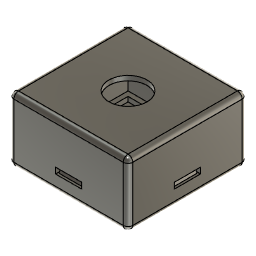
Button_case (Autodesk Fusion 360 design; units mm, degrees)
Autodesk Fusion 360 part; units mm, degrees
note: some values were not read from the file. Set by a fixed rule: which sketch regions a step uses.
sketch "Sketch1" plane through (0, 0, 0) normal (0, 0, 1) x (1, 0, 0)
  line L0 (0, 0) -> (50, 0)
  line L1 (50, 0) -> (50, 50)
  line L2 (50, 50) -> (0, 50)
  line L3 (0, 50) -> (0, 0)
  circle A0 centre (25, 25) radius 8
  line L4 (2, 48) -> (48, 48)
  line L5 (48, 48) -> (48, 2)
  line L6 (48, 2) -> (2, 2)
  line L7 (2, 2) -> (2, 48)
  constraint horizontal L0
  constraint vertical L1
  constraint horizontal L2
  constraint vertical L3
  constraint coincident L0.start L3.end
  constraint horizontal L4
  constraint vertical L5
  constraint horizontal L6
  constraint vertical L7
extrude "Extrude1" add sketch "Sketch1" along normal blind 2 contours L0 L1 L2 L3 | L4 L5 L6 L7 makes body 1
extrude "Extrude2" add sketch "Sketch1" against normal blind 23 contours L0 L1 L2 L3 bodies 1
fillet "Fillet1" radius 2 8 edges at (0, 25, 2) (25, 0, 2) (25, 50, 2) (50, 25, 2) (0, 0, -10.5) (50, 0, -10.5) (50, 50, -10.5) (0, 50, -10.5) on bodies 1
sketch "Sketch2" plane through (0, 0, -23) normal (0, 0, -1) x (1, 0, 0)
  arc A0 (50, -2) -> (48, 0) centre (48, -2) ccw
  line L0 (48, 0) -> (2, 0)
  arc A1 (2, 0) -> (0, -2) centre (2, -2) ccw
  line L1 (0, -2) -> (0, -48)
  arc A2 (0, -48) -> (2, -50) centre (2, -48) ccw
  line L2 (2, -50) -> (48, -50)
  arc A3 (48, -50) -> (50, -48) centre (48, -48) ccw
  line L3 (50, -48) -> (50, -2)
  line L4 (2, -2) -> (48, -2)
  line L5 (48, -2) -> (48, -48)
  line L6 (48, -48) -> (2, -48)
  line L7 (2, -48) -> (2, -2)
  line L8 (0, 0) -> (50, 0)
  line L9 (50, 0) -> (50, -50)
  line L10 (50, -50) -> (0, -50)
  line L11 (0, -50) -> (0, 0)
  line L12 (2, -2) -> (48, -2)
  line L13 (48, -2) -> (48, -48)
  line L14 (48, -48) -> (2, -48)
  line L15 (2, -48) -> (2, -2)
  line L16 (4, -46) -> (46, -46)
  line L17 (46, -46) -> (46, -4)
  line L18 (46, -4) -> (4, -4)
  line L19 (4, -4) -> (4, -46)
  constraint horizontal L8
  constraint vertical L9
  constraint horizontal L10
  constraint vertical L11
  constraint coincident L8.start L11.end
  constraint horizontal L12
  constraint vertical L13
  constraint horizontal L14
  constraint vertical L15
  constraint coincident A3.centre L5.end
  constraint coincident A1.centre L4.start
  constraint horizontal L16
  constraint vertical L17
  constraint horizontal L18
  constraint vertical L19
extrude "Extrude3" add sketch "Sketch2" along normal blind 2 separate body contours A0 L0 A1 L1 A2 L2 A3 L3 L8 L9 L10 L11 | L4 L5 L6 L7 L12 L13 L14 L15 | L16 L17 L18 L19 makes body 2
fillet "Fillet2" radius 2 8 edges at (50, 25, -25) (49.4142, 0.5858, -25) (25, 0, -25) (0.5858, 0.5858, -25) (0, 25, -25) (0.5858, 49.4142, -25) (25, 50, -25) (49.4142, 49.4142, -25) on bodies 2
extrude "Extrude4" add sketch "Sketch2" against normal blind 2 contours L4 L5 L6 L7 L12 L13 L14 L15 bodies 2
sketch "Sketch3" plane through (0, 0, -21) normal (0, 0, 1) x (-1, 0, 0)
  line L0 (-4, -4) -> (-4, -46)
  line L1 (-4, -46) -> (-46, -46)
  line L2 (-46, -46) -> (-46, -4)
  line L3 (-46, -4) -> (-4, -4)
  line L4 (-48, -48) -> (-2, -48)
  line L5 (-2, -48) -> (-2, -2)
  line L6 (-2, -2) -> (-48, -2)
  line L7 (-48, -2) -> (-48, -48)
  line L8 (-4, -30) -> (-2, -30)
  line L9 (-2, -30) -> (-2, -19.9838)
  line L10 (-2, -19.9838) -> (-4, -19.9838)
  line L11 (-4, -19.9838) -> (-4, -30)
  line L12 (-20, -46) -> (-30.0621, -46)
  line L13 (-30.0621, -46) -> (-30.0621, -48)
  line L14 (-30.0621, -48) -> (-20, -48)
  line L15 (-20, -48) -> (-20, -46)
  line L16 (-46, -30) -> (-48, -30)
  line L17 (-48, -30) -> (-48, -19.979)
  line L18 (-48, -19.979) -> (-46, -19.979)
  line L19 (-46, -19.979) -> (-46, -30)
  line L20 (-20, -4) -> (-30.0621, -4)
  line L21 (-30.0621, -4) -> (-30.0621, -2)
  line L22 (-30.0621, -2) -> (-20, -2)
  line L23 (-20, -2) -> (-20, -4)
  constraint horizontal L8
  constraint vertical L9
  constraint horizontal L10
  constraint vertical L11
  constraint coincident L5 L9.end
  constraint coincident L0 L8.start
  constraint horizontal L12
  constraint vertical L13
  constraint horizontal L14
  constraint vertical L15
  constraint coincident L4 L13.end
  constraint coincident L1 L12.start
  constraint horizontal L16
  constraint vertical L17
  constraint horizontal L18
  constraint vertical L19
  constraint coincident L7 L17.end
  constraint coincident L2 L16.start
  constraint horizontal L20
  constraint vertical L21
  constraint horizontal L22
  constraint vertical L23
  constraint coincident L6 L21.end
  constraint coincident L3 L20.start
extrude "Extrude5" add sketch "Sketch3" along normal blind 5 contours L0 L5 L8 L9 L10 L11 bodies 2
sketch "Sketch4" plane through (2, 0, 0) normal (-1, 0, 0) x (0, -1, 0)
  line L0 (-48, -23) -> (-2, -23)
  line L1 (-2, -23) -> (-2, -21)
  line L2 (-2, -21) -> (-19.9838, -21)
  line L3 (-19.9838, -21) -> (-19.9838, -16)
  line L4 (-19.9838, -16) -> (-30, -16)
  line L5 (-30, -16) -> (-30, -21)
  line L6 (-30, -21) -> (-48, -21)
  line L7 (-48, -21) -> (-48, -23)
  line L8 (-30, -16) -> (-19.9838, -16)
  line L9 (-19.9838, -16) -> (-19.9838, -18.5)
  line L10 (-19.9838, -18.5) -> (-30, -18.5)
  line L11 (-30, -18.5) -> (-30, -16)
  constraint horizontal L8
  constraint vertical L9
  constraint horizontal L10
  constraint vertical L11
  constraint midpoint L3 L9.end
  constraint coincident L4.end L5.start
extrude "Extrude6" add sketch "Sketch4" along normal blind 2 contours L3 L4 L5 L8 L9 L10 L11 bodies 2
sketch "Sketch5" plane through (0, 30, 0) normal (0, 1, 0) x (-1, 0, 0)
  line L0 (-4, -21) -> (-2, -21)
  line L1 (-2, -21) -> (-2, -18.5)
  line L2 (-2, -18.5) -> (0, -18.5)
  line L3 (0, -18.5) -> (0, -16)
  line L4 (0, -16) -> (-4, -16)
  line L5 (-4, -16) -> (-4, -21)
  line L6 (0, -18.5) -> (0, -17.5)
  line L7 (0, -17.5) -> (-2, -16)
  line L8 (0, -18.5) -> (-1, -18.5)
  line L9 (-1, -18.5) -> (-2, -16)
  constraint coincident L2.end L3.start
  constraint coincident L3 L6.end
  constraint perpendicular L2 L6
  constraint midpoint L4 L7.end
  constraint midpoint L2 L8.end
extrude "Extrude7" cut sketch "Sketch5" against normal blind 28 contours L3 L4 L7 bodies 2
copy_body "CopyPasteBodies1" bodies 2 makes body 3
move_body "Move1" bodies 3 to x (1, 0, 0) y (0, 1, 0) z (0, 0, 1) at (0, 0, 0)
combine "Combine1" operation cut target body 1 tool bodies 3
extrude "Extrude8" add sketch "Sketch3" along normal blind 5 contours L3 L6 L20 L21 L22 L23 | L1 L4 L12 L13 L14 L15 | L2 L7 L16 L17 L18 L19 bodies 2
sketch "Sketch6" plane through (0, 2, 0) normal (0, -1, 0) x (1, 0, 0)
  line L0 (2, -23) -> (48, -23)
  line L1 (48, -23) -> (48, -21)
  line L2 (48, -21) -> (30.0621, -21)
  line L3 (30.0621, -21) -> (30.0621, -16)
  line L4 (30.0621, -16) -> (20, -16)
  line L5 (20, -16) -> (20, -21)
  line L6 (20, -21) -> (2, -21)
  line L7 (2, -21) -> (2, -23)
  line L8 (20, -16) -> (30.0621, -16)
  line L9 (30.0621, -16) -> (30.0621, -18.5)
  line L10 (30.0621, -18.5) -> (20, -18.5)
  line L11 (20, -18.5) -> (20, -16)
  constraint horizontal L8
  constraint vertical L9
  constraint horizontal L10
  constraint vertical L11
  constraint midpoint L3 L9.end
  constraint coincident L4.end L5.start
extrude "Extrude9" add sketch "Sketch6" along normal blind 2 contours L3 L4 L5 L8 L9 L10 L11 bodies 2
sketch "Sketch7" plane through (20, 0, 0) normal (-1, 0, 0) x (0, -1, 0)
  line L0 (-4, -21) -> (-2, -21)
  line L1 (-2, -21) -> (-2, -18.5)
  line L2 (-2, -18.5) -> (0, -18.5)
  line L3 (0, -18.5) -> (0, -16)
  line L4 (0, -16) -> (-4, -16)
  line L5 (-4, -16) -> (-4, -21)
  line L6 (-2, -16) -> (0, -17.5)
  line L7 (0, -18.5) -> (-1, -18.5)
  line L8 (-2, -16) -> (-1, -18.5)
  constraint midpoint L4 L6.start
  constraint coincident L3 L6.end
  constraint coincident L2.end L3.start
  constraint midpoint L2 L7.end
extrude "Extrude10" cut sketch "Sketch7" against normal blind 42 contours L3 L4 L6 bodies 2
sketch "Sketch8" plane through (0, 48, 0) normal (0, 1, 0) x (-1, 0, 0)
  line L0 (-48, -23) -> (-2, -23)
  line L1 (-2, -23) -> (-2, -21)
  line L2 (-2, -21) -> (-20, -21)
  line L3 (-20, -21) -> (-20, -16)
  line L4 (-20, -16) -> (-30.0621, -16)
  line L5 (-30.0621, -16) -> (-30.0621, -21)
  line L6 (-30.0621, -21) -> (-48, -21)
  line L7 (-48, -21) -> (-48, -23)
  line L8 (-30.0621, -16) -> (-20, -16)
  line L9 (-20, -16) -> (-20, -18.5)
  line L10 (-20, -18.5) -> (-30.0621, -18.5)
  line L11 (-30.0621, -18.5) -> (-30.0621, -16)
  constraint horizontal L8
  constraint vertical L9
  constraint horizontal L10
  constraint vertical L11
  constraint midpoint L3 L9.end
  constraint coincident L4.end L5.start
extrude "Extrude11" add sketch "Sketch8" along normal blind 2 contours L3 L4 L5 L8 L9 L10 L11 bodies 2
sketch "Sketch9" plane through (30.0621, 0, 0) normal (1, 0, 0) x (0, 1, 0)
  line L0 (46, -21) -> (48, -21)
  line L1 (48, -21) -> (48, -18.5)
  line L2 (48, -18.5) -> (50, -18.5)
  line L3 (50, -18.5) -> (50, -16)
  line L4 (50, -16) -> (46, -16)
  line L5 (46, -16) -> (46, -21)
  line L6 (48, -16) -> (50, -17.5)
  line L7 (50, -18.5) -> (49, -18.5)
  line L8 (48, -16) -> (49, -18.5)
  constraint midpoint L4 L6.start
  constraint coincident L3 L6.end
  constraint coincident L2.end L3.start
  constraint midpoint L2 L7.end
extrude "Extrude12" cut sketch "Sketch9" against normal blind 37 contours L3 L4 L6 bodies 2
sketch "Sketch10" plane through (48, 0, 0) normal (1, 0, 0) x (0, 1, 0)
  line L0 (2, -23) -> (48, -23)
  line L1 (48, -23) -> (48, -21)
  line L2 (48, -21) -> (30, -21)
  line L3 (30, -21) -> (30, -16)
  line L4 (30, -16) -> (19.979, -16)
  line L5 (19.979, -16) -> (19.979, -21)
  line L6 (19.979, -21) -> (2, -21)
  line L7 (2, -21) -> (2, -23)
  line L8 (19.979, -16) -> (30, -16)
  line L9 (30, -16) -> (30, -18.5)
  line L10 (30, -18.5) -> (19.979, -18.5)
  line L11 (19.979, -18.5) -> (19.979, -16)
  constraint horizontal L8
  constraint vertical L9
  constraint horizontal L10
  constraint vertical L11
  constraint midpoint L3 L9.end
  constraint coincident L4.end L5.start
extrude "Extrude13" add sketch "Sketch10" along normal blind 2 contours L3 L4 L5 L8 L9 L10 L11 bodies 2
sketch "Sketch11" plane through (0, 19.979, 0) normal (0, -1, 0) x (1, 0, 0)
  line L0 (46, -21) -> (48, -21)
  line L1 (48, -21) -> (48, -18.5)
  line L2 (48, -18.5) -> (50, -18.5)
  line L3 (50, -18.5) -> (50, -16)
  line L4 (50, -16) -> (46, -16)
  line L5 (46, -16) -> (46, -21)
  line L6 (48, -16) -> (50, -17.5)
  line L7 (50, -18.5) -> (49, -18.5)
  line L8 (49, -16.75) -> (49, -18.5)
  line L9 (48, -16) -> (49, -18.5)
  constraint midpoint L4 L6.start
  constraint coincident L3 L6.end
  constraint coincident L2.end L3.start
  constraint midpoint L2 L7.end
  constraint midpoint L6 L8.start
extrude "Extrude14" cut sketch "Sketch11" against normal blind 23 contours L3 L4 L6 bodies 2
copy_body "CopyPasteBodies2" bodies 2 makes body 4
move_body "Move2" bodies 4 to x (1, 0, 0) y (0, 1, 0) z (0, 0, 1) at (0, 0, 0)
combine "Combine2" operation cut target body 1 tool bodies 4
sketch "Sketch12" plane through (0, 0, 0) normal (-1, 0, 0) x (0, -1, 0)
  line L0 (-30, -17.5) -> (-19.9838, -17.5)
  line L1 (-19.9838, -17.5) -> (-19.9838, -18.5)
  line L2 (-19.9838, -18.5) -> (-30, -18.5)
  line L3 (-30, -18.5) -> (-30, -17.5)
  line L4 (-2, -23) -> (-2, 0)
  line L5 (-2, 0) -> (-48, 0)
  line L6 (-48, 0) -> (-48, -23)
  line L7 (-48, -23) -> (-2, -23)
  line L8 (-30, -18.5) -> (-30.5, -18.5)
  line L9 (-30.5, -18.5) -> (-30.5, -19)
  line L10 (-19.9838, -18.5) -> (-19.5, -18.5)
  line L11 (-19.5, -18.5) -> (-19.5, -19)
  line L12 (-19.5, -19) -> (-30.5, -19)
  line L13 (-30.5, -19) -> (-30.5, -16)
  line L14 (-30.5, -16) -> (-19.5, -16)
  line L15 (-19.5, -16) -> (-19.5, -18.5)
  line L16 (-19.9838, -18.5) -> (-19.5, -18.5)
  line L17 (-30, -18.5) -> (-30.5, -18.5)
  constraint coincident L2.end L3.start
  constraint perpendicular L3 L8
  constraint perpendicular L8 L9
  constraint coincident L1.end L2.start
  constraint perpendicular L1 L10
  constraint perpendicular L10 L11
  constraint perpendicular L8 L13
  constraint perpendicular L13 L14
  constraint perpendicular L10 L15
extrude "Extrude15" cut sketch "Sketch12" against normal blind 84 contours L0 L1 L3 L8 L10 L13 L14 L15 L16 L17 bodies 1
sketch "Sketch13" plane through (0, 50, 0) normal (0, 1, 0) x (-1, 0, 0)
  line L0 (-30.0621, -17.5) -> (-20, -17.5)
  line L1 (-20, -17.5) -> (-20, -18.5)
  line L2 (-20, -18.5) -> (-30.0621, -18.5)
  line L3 (-30.0621, -18.5) -> (-30.0621, -17.5)
  line L4 (-48, 0) -> (-48, -23)
  line L5 (-48, -23) -> (-2, -23)
  line L6 (-2, -23) -> (-2, 0)
  line L7 (-2, 0) -> (-48, 0)
  line L8 (-30.0621, -18.5) -> (-30.5, -18.5)
  line L9 (-30.5, -18.5) -> (-30.5, -15.5)
  line L10 (-30.5, -15.5) -> (-19.5, -15.5)
  line L11 (-19.5, -15.5) -> (-19.5, -18.5)
  line L12 (-20, -18.5) -> (-19.5, -18.5)
  line L13 (-30.5, -15.5) -> (-30.5, -16)
  line L14 (-19.5, -16) -> (-30.5, -16)
  line L15 (-25, 2) -> (-25, -25)
  line L16 (-25, -25) -> (-25, -11.5)
  ellipse E0 centre (-25, -11) end of major axis (-22, -11) minor radius 2
  line L17 (-28, -11) -> (-22, -11)
  line L18 (-25, -13) -> (-25, -9)
  constraint coincident L2.end L3.start
  constraint perpendicular L3 L8
  constraint perpendicular L8 L9
  constraint perpendicular L9 L10
  constraint perpendicular L10 L11
  constraint coincident L1.end L2.start
  constraint perpendicular L11 L12
  constraint coincident L9 L13.end
  constraint coincident L11 L14.start
  constraint perpendicular L13 L14
  constraint perpendicular L5 L15
  constraint midpoint L15 L16.end
  constraint perpendicular L10 L16
  constraint coincident L15 E0.centre
  constraint perpendicular L15 L17
  constraint coincident E0 L17.start
  constraint coincident E0 L17.end
  constraint coincident E0 L18.start
  constraint coincident E0 L18.end
extrude "Extrude16" cut sketch "Sketch13" against normal blind 160 contours L0 L3 L8 L9 L14 L15 L16 | L0 L1 L11 L12 L14 L15 L16 bodies 1
extrude "Extrude17" cut sketch "Sketch13" against normal blind 4 contours L15 L16 E0 L17 L18 | L15 L16 E0 L17 L18 | L15 E0 L17 L18 | L15 E0 L17 L18 bodies 1
extrude "Extrude18" cut sketch "Sketch11" against normal blind 23 contours L6 L8 L9 | L2 L3 L6 L7 L8 bodies 2
extrude "Extrude19" cut sketch "Sketch9" against normal blind 16 contours L2 L3 L6 L7 L8 bodies 2
extrude "Extrude20" cut sketch "Sketch7" against normal blind 42 contours L2 L3 L6 L7 L8 bodies 2
extrude "Extrude21" cut sketch "Sketch5" against normal blind 11 contours L2 L3 L6 L7 L8 L9 bodies 2
